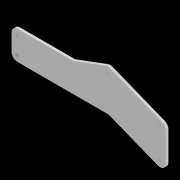
# Autodesk Inventor part: switchback-secondary-cover
Saved by Autodesk Inventor 2020 (Build 240168000, 168)
## iProperties
Created: 2020-01-08
Part Number: switchback-secondary-cover
Material: Generic
Document SubType Name: Modeling
Designer: valer
Density: 1 g/cm^3
Appearance: Default
Author: valer
Autodesk Inventor part; units mm, degrees
ref_plane "YZ Plane" through (0, 0, 0) normal (1, 0, 0) x (0, 1, 0)
ref_plane "XZ Plane" through (0, 0, 0) normal (0, 1, 0) x (-1, 0, 0)
ref_plane "XY Plane" through (0, 0, 0) normal (0, 0, 1) x (1, 0, 0)
sketch "Profile" plane through (0, 0, 0) normal (0, 0, 1) x (1, 0, 0)
  circle A0 centre (1024.5892, 81.5101) radius 1.27
  circle A1 centre (869.1584, 103.2274) radius 1.27
  circle A2 centre (869.1584, 121.6106) radius 1.27
  circle A3 centre (967.608, 135.3677) radius 1.27
  circle A4 centre (1024.5892, 112.7794) radius 1.27
  line L0 (963.5286, 137.2438) -> (964.6303, 134.266)
  arc A5 (964.6303, 134.266) -> (970.5595, 134.1976) centre (967.608, 135.3677) ccw
  line L1 (970.5595, 134.1976) -> (971.7296, 137.1492)
  line L2 (1022.8077, 116.901) -> (971.7296, 137.1492)
  line L3 (1022.8077, 116.901) -> (1021.6376, 113.9494)
  arc A6 (1021.6376, 113.9494) -> (1024.5892, 109.6044) centre (1024.5892, 112.7794) ccw
  line L4 (1024.5892, 109.6044) -> (1027.7642, 109.6044)
  line L5 (1027.7642, 84.6851) -> (1027.7642, 109.6044)
  line L6 (1027.7642, 84.6851) -> (1024.5892, 84.6851)
  arc A7 (1024.5892, 84.6851) -> (1021.6376, 82.6802) centre (1024.5892, 81.5101) ccw
  line L7 (1021.6376, 82.6802) -> (1020.4676, 79.7286)
  line L8 (970.7004, 99.4571) -> (1020.4676, 79.7286)
  arc A8 (970.7004, 99.4571) -> (967.5834, 100.0524) centre (967.5834, 91.5942) ccw
  line L9 (872.3334, 100.0524) -> (967.5834, 100.0524)
  line L10 (872.3334, 100.0524) -> (872.3334, 103.2274)
  arc A9 (872.3334, 103.2274) -> (869.1584, 106.4024) centre (869.1584, 103.2274) ccw
  line L11 (869.1584, 106.4024) -> (865.9834, 106.4024)
  line L12 (865.9834, 118.4356) -> (865.9834, 106.4024)
  line L13 (865.9834, 118.4356) -> (869.1584, 118.4356)
  arc A10 (869.1584, 118.4356) -> (872.3334, 121.6106) centre (869.1584, 121.6106) ccw
  line L14 (872.3334, 121.6106) -> (872.3334, 124.7856)
  line L15 (929.2861, 124.7856) -> (872.3334, 124.7856)
  arc A11 (929.2861, 124.7856) -> (930.3878, 124.9829) centre (929.2861, 127.9606) ccw
  line L16 (963.5286, 137.2438) -> (930.3878, 124.9829)
  line L17 (869.1584, 127.9606) -> (929.2861, 127.9606)
  arc A12 (869.1584, 127.9606) -> (862.8084, 121.6106) centre (869.1584, 121.6106) ccw
  line L18 (862.8084, 103.2274) -> (862.8084, 121.6106)
  arc A13 (862.8084, 103.2274) -> (869.1584, 96.8774) centre (869.1584, 103.2274) ccw
  line L19 (967.5834, 96.8774) -> (869.1584, 96.8774)
  arc A14 (969.5304, 96.5056) -> (967.5834, 96.8774) centre (967.5834, 91.5942) ccw
  line L20 (1022.2491, 75.607) -> (969.5304, 96.5056)
  arc A15 (1022.2491, 75.607) -> (1030.9392, 81.5101) centre (1024.5892, 81.5101) ccw
  line L21 (1030.9392, 112.7794) -> (1030.9392, 81.5101)
  arc A16 (1030.9392, 112.7794) -> (1026.9292, 118.6825) centre (1024.5892, 112.7794) ccw
  line L22 (969.9481, 141.2708) -> (1026.9292, 118.6825)
  arc A17 (969.9481, 141.2708) -> (965.4047, 141.3232) centre (967.608, 135.3677) ccw
  line L23 (929.2861, 127.9606) -> (965.4047, 141.3232)
  point P0 (0, 0)
  constraints: 48 end point, 26 point on circle, 18 centre point
extrude "ProfileFeature" add sketch "Profile" along normal blind 2.54 contours L0 A5 L1 L2 L3 A6 L4 L5 L6 A7 L7 L8 A8 L9 L10 A9 L11 L12 L13 A10 L14 L15 A11 L16 | L17 L23 A17 L22 A16 L21 A15 L20 A14 L19 A13 L18 A12
body "Solid1"
